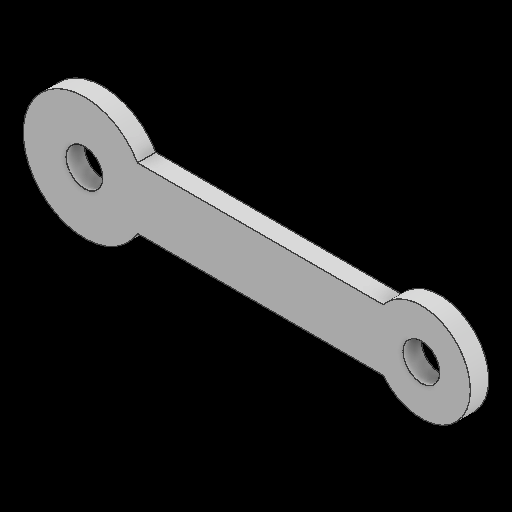
# Autodesk Inventor part: LegChainTensionerArm
Saved by Autodesk Inventor 2025.2 (Build 292293000, 293)
## iProperties
Created: 2026-01-19
Part Number: LegChainTensionerArm
Material: Generic
Document SubType Name: Sheet Metal
Designer: valer
Density: 1 g/cm^3
Sheet Metal Rule: Default_mm
Appearance: Default
Author: valer
Autodesk Inventor part; units mm, degrees
ref_plane "YZ Plane" through (0, 0, 0) normal (1, 0, 0) x (0, 1, 0)
ref_plane "XZ Plane" through (0, 0, 0) normal (0, 1, 0) x (-1, 0, 0)
ref_plane "XY Plane" through (0, 0, 0) normal (0, 0, 1) x (1, 0, 0)
sketch "Base" plane through (0, 0, 0) normal (0, 0, 1) x (1, 0, 0)
  circle A0 centre (0, 0) radius 10
  line L0 (0, 0) -> (55, 0) construction
  circle A1 centre (55, 0) radius 8
  line L1 (8.6603, 5) -> (48.755, 5)
  line L2 (48.755, 5) -> (48.755, -5)
  line L3 (48.755, -5) -> (8.6603, -5)
  line L4 (8.6603, -5) -> (8.6603, 5)
  circle A2 centre (55, 0) radius 3
  circle A3 centre (0, 0) radius 3
  point P0 (8.6603, 0)
  point P1 (8.6603, -5)
  dimension "d0" = 20
  dimension "d2" = 16
  dimension "d1" = 55
  dimension "d3" = 10
  dimension "d4" = 6
  dimension "d5" = 6
  measures "d1" distance of L0.start L0.end
  measures "d3" distance of L3.end L1.start
  measures "d4" diameter of A2
  measures "d5" diameter of A3
extrude "Plate1" add sketch "Base" along normal blind 3
equation "\"d6\" = Thickness"
equation "\"BendRadius\" = Thickness"
equation "\"BendReliefWidth\" = Thickness"
equation "\"BendReliefDepth\" = 0.5 * Thickness"
equation "\"CornerReliefSize\" = 4 * Thickness"
equation "\"MinimumRemnant\" = 2 * Thickness"
equation "\"TransitionRadius\" = BendRadius"
equation "\"JacobiRadiusSize\" = BendRadius"
equation "\"GapSize\" = Thickness"
equation "\"Thickness\" = 3"
body "Solid1"
